Autodesk Fusion 360 part; units mm, degrees
(part 2 of 3)
  constraint coincident L1 L360.end
  constraint perpendicular L1 L360
  constraint midpoint L6 L361.start
  constraint coincident L3 L361.end
  constraint perpendicular L3 L361
  constraint equal L360 L361
  constraint midpoint L4 L362.start
  constraint perpendicular L2 L362
  constraint coincident L2 L362.end
  constraint coincident A356.centre L363.start
  constraint coincident L2 L363.end
  constraint perpendicular L2 L363
  constraint coincident L3 L364.end
  constraint perpendicular L3 L364
  constraint equal L363 L364
  constraint midpoint L2 L365.start
  constraint perpendicular L2 L365
  constraint midpoint L3 L366.start
  constraint perpendicular L3 L366
  constraint symmetric A356 L365 A357
  constraint symmetric A356 L366 A358
  constraint symmetric L366 A357 A359
  constraint equal A2 A52
  constraint equal A2 A3
  constraint tangent L5 A3
  constraint tangent L7 A3
  constraint tangent L5 A2
  constraint tangent L6 A2
  constraint vertical L7.start L59.start
  constraint tangent L4 A1
  constraint vertical A3.centre A53.centre
  constraint tangent L7 A1
  constraint tangent L6 A0
  constraint vertical A2.centre A52.centre
  constraint tangent L4 A0
  constraint horizontal L4
  constraint vertical L6
  constraint equal A0 A1
  constraint equal A1 A3
  constraint equal L6 L58
  constraint vertical A6.centre A60.centre
  constraint horizontal A3.centre A6.centre
  constraint horizontal A7.centre A10.centre
  constraint horizontal A11.centre A14.centre
  constraint horizontal A15.centre A18.centre
  constraint horizontal A19.centre A22.centre
  constraint horizontal A23.centre A26.centre
  constraint horizontal A27.centre A30.centre
  constraint horizontal A31.centre A34.centre
  constraint horizontal A35.centre A38.centre
  constraint horizontal A39.centre A42.centre
  constraint horizontal A43.centre A46.centre
  constraint horizontal A47.centre A50.centre
  constraint tangent L8 A4
  constraint tangent L10 A4
  constraint tangent L10 A6
  constraint tangent L9 A6
  constraint tangent L9 A7
  constraint tangent L11 A7
  constraint tangent L8 A5
  constraint tangent L11 A5
  constraint horizontal L8
  constraint vertical L10
  constraint horizontal L9
  constraint vertical L11
  constraint equal A4 A5
  constraint equal A6 A7
  constraint equal A4 A6
  constraint horizontal L12
  constraint vertical L14
  constraint horizontal L13
  constraint vertical L15
  constraint equal A8 A9
  constraint equal A8 A10
  constraint equal A10 A11
  constraint tangent L14 A10
  constraint tangent L13 A10
  constraint tangent L13 A11
  constraint tangent L15 A11
  constraint tangent L15 A9
  constraint tangent L12 A9
  constraint tangent L12 A8
  constraint tangent L14 A8
  constraint equal L8 L10
  constraint equal L12 L14
  constraint equal L16 L18
  constraint horizontal L16
  constraint vertical L18
  constraint horizontal L17
  constraint vertical L19
  constraint tangent L16 A13
  constraint tangent L19 A13
  constraint tangent L16 A12
  constraint tangent L18 A12
  constraint tangent L18 A14
  constraint tangent L17 A14
  constraint tangent L17 A15
  constraint tangent L19 A15
  constraint equal A12 A13
  constraint equal A12 A14
  constraint equal A14 A15
  constraint horizontal L20
  constraint horizontal L21
  constraint vertical L23
  constraint horizontal L24
  constraint vertical L26
  constraint vertical L22
  constraint horizontal L25
  constraint vertical L27
  constraint horizontal L28
  constraint vertical L30
  constraint vertical L31
  constraint horizontal L29
  constraint horizontal L32
  constraint horizontal L33
  constraint vertical L35
  constraint vertical L34
  constraint horizontal L36
  constraint horizontal L37
  constraint vertical L38
  constraint vertical L39
  constraint vertical L42
  constraint horizontal L40
  constraint vertical L43
  constraint horizontal L41
  constraint horizontal L45
  constraint vertical L46
  constraint horizontal L44
  constraint vertical L47
  constraint horizontal L48
  constraint vertical L50
  constraint horizontal L49
  constraint vertical L51
  constraint vertical L54
  constraint horizontal L52
  constraint vertical L55
  constraint horizontal L53
  constraint tangent L24 A20
  constraint tangent L26 A22
  constraint tangent L26 A20
  constraint tangent L25 A22
  constraint tangent L25 A23
  constraint tangent L24 A21
  constraint tangent L27 A21
  constraint tangent L27 A23
  constraint tangent L20 A16
  constraint tangent L22 A16
  constraint tangent L22 A18
  constraint tangent L21 A18
  constraint tangent L21 A19
  constraint tangent L23 A19
  constraint tangent L23 A17
  constraint tangent L20 A17
  constraint equal L20 L22
  constraint equal L24 L26
  constraint equal L28 L30
  constraint equal L32 L34
  constraint equal L36 L38
  constraint equal L40 L42
  constraint equal L44 L46
  constraint equal L48 L50
  constraint equal L52 L54
  constraint equal A16 A17
  constraint equal A16 A18
  constraint equal A17 A19
  constraint equal A20 A21
  constraint equal A21 A23
  constraint equal A22 A23
  constraint equal A24 A25
  constraint equal A25 A27
  constraint equal A26 A27
  constraint equal A26 A28
  constraint equal A28 A29
  constraint equal A29 A31
  constraint equal A30 A31
  constraint equal A30 A32
  constraint equal A32 A33
  constraint equal A33 A35
  constraint equal A34 A35
  constraint equal A34 A36
  constraint equal A36 A37
  constraint equal A37 A39
  constraint equal A38 A39
  constraint equal A38 A40
  constraint equal A40 A41
  constraint equal A41 A43
  constraint equal A42 A43
  constraint equal A42 A46
  constraint equal A44 A46
  constraint equal A44 A45
  constraint equal A45 A47
  constraint equal A47 A50
  constraint equal A48 A50
  constraint equal A48 A49
  constraint equal A49 A51
  constraint tangent L28 A24
  constraint tangent L30 A24
  constraint tangent L30 A26
  constraint tangent L29 A26
  constraint tangent L29 A27
  constraint tangent L31 A27
  constraint tangent L28 A25
  constraint tangent L31 A25
  constraint tangent L32 A28
  constraint tangent L34 A28
  constraint tangent L34 A30
  constraint tangent L33 A30
  constraint tangent L32 A29
  constraint tangent L35 A29
  constraint tangent L36 A32
  constraint tangent L38 A32
  constraint tangent L35 A31
  constraint tangent L38 A34
  constraint tangent L33 A31
  constraint tangent L37 A34
  constraint tangent L36 A33
  constraint tangent L39 A33
  constraint tangent L39 A35
  constraint tangent L37 A35
  constraint tangent L40 A36
  constraint tangent L42 A36
  constraint tangent L40 A37
  constraint tangent L43 A37
  constraint tangent L43 A39
  constraint tangent L41 A39
  constraint tangent L42 A38
  constraint tangent L41 A38
  constraint tangent L44 A40
  constraint tangent L44 A41
  constraint tangent L47 A41
  constraint tangent L47 A43
  constraint tangent L45 A43
  constraint tangent L46 A42
  constraint tangent L45 A42
  constraint tangent L46 A40
  constraint tangent L50 A46
  constraint tangent L49 A46
  constraint tangent L49 A47
  constraint tangent L51 A47
  constraint tangent L48 A44
  constraint tangent L50 A44
  constraint tangent L48 A45
  constraint tangent L51 A45
  constraint tangent L52 A48
  constraint tangent L54 A48
  constraint tangent L54 A50
  constraint tangent L53 A50
  constraint tangent L53 A51
  constraint tangent L55 A51
  constraint tangent L55 A49
  constraint tangent L52 A49
  constraint equal L8 L12
  constraint equal L12 L16
  constraint equal L16 L20
  constraint equal L20 L24
  constraint equal L24 L28
  constraint equal L28 L32
  constraint equal L32 L36
  constraint equal L36 L40
  constraint equal L40 L44
  constraint equal L44 L48
  constraint equal L48 L52
  constraint equal A5 A8
  constraint equal A9 A12
  constraint equal A13 A16
  constraint equal A17 A20
  constraint equal A1 A4
  constraint equal L7 L10
  constraint midpoint L11 L367.start
  constraint midpoint L14 L367.end
  constraint midpoint L15 L368.start
  constraint midpoint L18 L368.end
  constraint midpoint L19 L369.start
  constraint midpoint L22 L369.end
  constraint parallel L368 L369
  constraint midpoint L27 L370.start
  constraint midpoint L30 L370.end
  constraint midpoint L31 L371.start
  constraint midpoint L34 L371.end
  constraint midpoint L35 L372.start
  constraint midpoint L38 L372.end
  constraint midpoint L43 L373.start
  constraint midpoint L46 L373.end
  constraint midpoint L47 L374.start
  constraint midpoint L50 L374.end
  constraint midpoint L51 L375.start
  constraint midpoint L54 L375.end
  constraint equal L374 L375
  constraint equal L373 L374
  constraint equal L372 L373
  constraint midpoint L59 L376.start
  constraint midpoint L62 L376.end
  constraint equal L375 L376
  constraint equal L371 L372
  constraint equal L370 L371
  constraint equal L369 L370
  constraint equal L367 L368
  constraint equal L368 L376
  constraint midpoint L39 L377.start
  constraint midpoint L42 L377.end
  constraint midpoint L23 L378.start
  constraint midpoint L26 L378.end
  constraint equal L377 L378
  constraint equal A21 A24
  constraint horizontal L379
  constraint perpendicular L379 L380
  constraint parallel L379 L381
  constraint parallel L380 L382
  constraint coincident L383 P1
  constraint coincident L384 P1
  constraint equal L379 L382
  constraint midpoint L55 P2
  constraint horizontal P1 P2
  constraint coincident P1 P0
  constraint horizontal L360.start P5
  constraint midpoint L120 P4
  constraint vertical P5 P4
  constraint horizontal L385
  constraint perpendicular L385 L386
  constraint parallel L385 L387
  constraint parallel L386 L388
  constraint coincident L389 P5
  constraint coincident L390 P5
  constraint coincident P5 P3
  constraint equal L385 L388
  constraint midpoint L52 P6
  constraint vertical P1 P6
  constraint horizontal L391
  constraint perpendicular L391 L392
  constraint parallel L391 L393
  constraint parallel L392 L394
  constraint coincident L395 P7
  constraint coincident L396 P7
  constraint equal L379 L391
  constraint equal L391 L392
  constraint vertical L362.start P7
  constraint horizontal L361.start P7
  constraint midpoint L56 P8
  constraint midpoint L58 P9
  constraint horizontal L397
  constraint perpendicular L397 L398
  constraint parallel L397 L399
  constraint parallel L398 L400
  constraint coincident L401 P10
  constraint coincident L402 P10
  constraint vertical P8 P10
  constraint horizontal P9 P10
  constraint equal L397 L400
  constraint equal L393 L397
  measures "d28" distance of L0.start L2.end
  measures "d29" distance of L1.end L2.end
  measures "d32" diameter of A356
  measures "d33" distance of A356.centre L363.end
  measures "d35" distance of L0 L313
  measures "d39" distance of L379.start L379.end
  measures "d40" distance of L385.start L386.start
  measures "d41" distance of L382 L386
  measures "d42" distance of L393 L397
  measures "d43" diameter of A360
extrude "Extrude1" add sketch "plate-2026-01-07T20_54_01.375Z" along normal blind 1.5
fillet "Fillet1" radius 2.5 4 edges at (-11.2624, 12.475, 0.75) (-11.2624, -135.013, 0.75) (318.4436, -135.013, 0.75) (318.4436, 12.475, 0.75)
sketch "Sketch2" plane through (0, 0, 1.5) normal (0, 0, 1) x (-1, 0, 0)
  line L0 (-21.154, 19.2163) -> (-45.304, 19.2163) construction
  line L1 (-45.304, 19.2163) -> (-45.304, 5.2163) construction
  line L2 (-45.304, 5.2163) -> (-21.154, 5.2163) construction
  line L3 (-21.154, 5.2163) -> (-21.154, 19.2163) construction
  arc A0 (-88.75, 50.15) -> (-88.25, 50.65) centre (-88.75, 50.65) ccw
  line L4 (-88.75, 50.15) -> (-101.75, 50.15)
  arc A1 (-102.25, 50.65) -> (-101.75, 50.15) centre (-101.75, 50.65) ccw
  line L5 (-102.25, 50.65) -> (-102.25, 63.65)
  arc A2 (-101.75, 64.15) -> (-102.25, 63.65) centre (-101.75, 63.65) ccw
  line L6 (-101.75, 64.15) -> (-88.75, 64.15)
  arc A3 (-88.25, 63.65) -> (-88.75, 64.15) centre (-88.75, 63.65) ccw
  line L7 (-88.25, 63.65) -> (-88.25, 50.65)
  arc A4 (-269.7253, 7.287) -> (-269.2252, 7.787) centre (-269.7253, 7.787) ccw
  line L8 (-269.7253, 7.287) -> (-282.7252, 7.287)
  arc A5 (-283.2253, 7.787) -> (-282.7252, 7.287) centre (-282.7252, 7.787) ccw
  line L9 (-283.2253, 7.787) -> (-283.2253, 20.787)
  arc A6 (-282.7252, 21.287) -> (-283.2253, 20.787) centre (-282.7252, 20.787) ccw
  line L10 (-282.7252, 21.287) -> (-269.7253, 21.287)
  arc A7 (-269.2253, 20.787) -> (-269.7253, 21.287) centre (-269.7253, 20.787) ccw
  line L11 (-269.2253, 20.787) -> (-269.2252, 7.787)
  arc A8 (-107.8, 50.15) -> (-107.3, 50.65) centre (-107.8, 50.65) ccw
  line L12 (-107.8, 50.15) -> (-120.8, 50.15)
  arc A9 (-121.3, 50.65) -> (-120.8, 50.15) centre (-120.8, 50.65) ccw
  line L13 (-121.3, 50.65) -> (-121.3, 63.65)
  arc A10 (-120.8, 64.15) -> (-121.3, 63.65) centre (-120.8, 63.65) ccw
  line L14 (-120.8, 64.15) -> (-107.8, 64.15)
  arc A11 (-107.3, 63.65) -> (-107.8, 64.15) centre (-107.8, 63.65) ccw
  line L15 (-107.3, 63.65) -> (-107.3, 50.65)
  arc A12 (-207.8125, 69.2) -> (-207.3125, 69.7) centre (-207.8125, 69.7) ccw
  line L16 (-207.8125, 69.2) -> (-220.8125, 69.2)
  arc A13 (-221.3125, 69.7) -> (-220.8125, 69.2) centre (-220.8125, 69.7) ccw
  line L17 (-221.3125, 69.7) -> (-221.3125, 82.7)
  arc A14 (-220.8125, 83.2) -> (-221.3125, 82.7) centre (-220.8125, 82.7) ccw
  line L18 (-220.8125, 83.2) -> (-207.8125, 83.2)
  arc A15 (-207.3125, 82.7) -> (-207.8125, 83.2) centre (-207.8125, 82.7) ccw
  line L19 (-207.3125, 82.7) -> (-207.3125, 69.7)
  arc A16 (-203.05, 50.15) -> (-202.55, 50.65) centre (-203.05, 50.65) ccw
  line L20 (-203.05, 50.15) -> (-216.05, 50.15)
  arc A17 (-216.55, 50.65) -> (-216.05, 50.15) centre (-216.05, 50.65) ccw
  line L21 (-216.55, 50.65) -> (-216.55, 63.65)
  arc A18 (-216.05, 64.15) -> (-216.55, 63.65) centre (-216.05, 63.65) ccw
  line L22 (-216.05, 64.15) -> (-203.05, 64.15)
  arc A19 (-202.55, 63.65) -> (-203.05, 64.15) centre (-203.05, 63.65) ccw
  line L23 (-202.55, 63.65) -> (-202.55, 50.65)
  arc A20 (-6.4933, 89.25) -> (-5.9933, 89.75) centre (-6.4932, 89.75) ccw
  line L24 (-6.4933, 89.25) -> (-12.4932, 89.25)
  arc A21 (-12.9933, 89.75) -> (-12.4932, 89.25) centre (-12.4932, 89.75) ccw
  line L25 (-12.9932, 89.75) -> (-12.9933, 103.75)
  arc A22 (-12.4932, 104.25) -> (-12.9933, 103.75) centre (-12.4932, 103.75) ccw
  line L26 (-12.4932, 104.25) -> (-6.4932, 104.25)
  arc A23 (-5.9932, 103.75) -> (-6.4932, 104.25) centre (-6.4933, 103.75) ccw
  line L27 (-5.9932, 103.75) -> (-5.9933, 89.75)
  arc A24 (-291.1562, 31.1) -> (-290.6562, 31.6) centre (-291.1563, 31.6) ccw
  line L28 (-291.1562, 31.1) -> (-304.1562, 31.1)
  arc A25 (-304.6562, 31.6) -> (-304.1562, 31.1) centre (-304.1563, 31.6) ccw
  line L29 (-304.6562, 31.6) -> (-304.6562, 44.6)
  arc A26 (-304.1562, 45.1) -> (-304.6563, 44.6) centre (-304.1563, 44.6) ccw
  line L30 (-304.1562, 45.1) -> (-291.1562, 45.1)
  arc A27 (-290.6562, 44.6) -> (-291.1563, 45.1) centre (-291.1562, 44.6) ccw
  line L31 (-290.6562, 44.6) -> (-290.6562, 31.6)
  arc A28 (-188.7625, 69.2) -> (-188.2625, 69.7) centre (-188.7625, 69.7) ccw
  line L32 (-188.7625, 69.2) -> (-201.7625, 69.2)
  arc A29 (-202.2625, 69.7) -> (-201.7625, 69.2) centre (-201.7625, 69.7) ccw
  line L33 (-202.2625, 69.7) -> (-202.2625, 82.7)
  arc A30 (-201.7625, 83.2) -> (-202.2625, 82.7) centre (-201.7625, 82.7) ccw
  line L34 (-201.7625, 83.2) -> (-188.7625, 83.2)
  arc A31 (-188.2625, 82.7) -> (-188.7625, 83.2) centre (-188.7625, 82.7) ccw
  line L35 (-188.2625, 82.7) -> (-188.2625, 69.7)
  arc A32 (-36.3625, 69.2) -> (-35.8625, 69.7) centre (-36.3625, 69.7) ccw
  line L36 (-36.3625, 69.2) -> (-49.3625, 69.2)
  arc A33 (-49.8625, 69.7) -> (-49.3625, 69.2) centre (-49.3625, 69.7) ccw
  line L37 (-49.8625, 69.7) -> (-49.8625, 82.7)
  arc A34 (-49.3625, 83.2) -> (-49.8625, 82.7) centre (-49.3625, 82.7) ccw
  line L38 (-49.3625, 83.2) -> (-36.3625, 83.2)
  arc A35 (-35.8625, 82.7) -> (-36.3625, 83.2) centre (-36.3625, 82.7) ccw
  line L39 (-35.8625, 82.7) -> (-35.8625, 69.7)
  arc A36 (-169.7125, 69.2) -> (-169.2125, 69.7) centre (-169.7125, 69.7) ccw
  line L40 (-169.7125, 69.2) -> (-182.7125, 69.2)
  arc A37 (-183.2125, 69.7) -> (-182.7125, 69.2) centre (-182.7125, 69.7) ccw
  line L41 (-183.2125, 69.7) -> (-183.2125, 82.7)
  arc A38 (-182.7125, 83.2) -> (-183.2125, 82.7) centre (-182.7125, 82.7) ccw
  line L42 (-182.7125, 83.2) -> (-169.7125, 83.2)
  arc A39 (-169.2125, 82.7) -> (-169.7125, 83.2) centre (-169.7125, 82.7) ccw
  line L43 (-169.2125, 82.7) -> (-169.2125, 69.7)
  arc A40 (-164.9501, 7.287) -> (-164.4501, 7.787) centre (-164.9501, 7.787) ccw
  line L44 (-164.9501, 7.287) -> (-177.9501, 7.287)
  arc A41 (-178.4501, 7.787) -> (-177.9501, 7.287) centre (-177.9501, 7.787) ccw
  line L45 (-178.4501, 7.787) -> (-178.4501, 20.787)
  arc A42 (-177.9501, 21.287) -> (-178.4501, 20.787) centre (-177.9501, 20.787) ccw
  line L46 (-177.9501, 21.287) -> (-164.9501, 21.287)
  arc A43 (-164.4501, 20.787) -> (-164.9501, 21.287) centre (-164.9501, 20.787) ccw
  line L47 (-164.4501, 20.787) -> (-164.4501, 7.787)
  arc A44 (-212.575, 31.1) -> (-212.075, 31.6) centre (-212.575, 31.6) ccw
  line L48 (-212.575, 31.1) -> (-225.575, 31.1)
  arc A45 (-226.075, 31.6) -> (-225.575, 31.1) centre (-225.575, 31.6) ccw
  line L49 (-226.075, 31.6) -> (-226.075, 44.6)
  arc A46 (-225.575, 45.1) -> (-226.075, 44.6) centre (-225.575, 44.6) ccw
  line L50 (-225.575, 45.1) -> (-212.575, 45.1)
  arc A47 (-212.075, 44.6) -> (-212.575, 45.1) centre (-212.575, 44.6) ccw
  line L51 (-212.075, 44.6) -> (-212.075, 31.6)
  arc A48 (-275.638, 32.1) -> (-275.138, 32.6) centre (-275.638, 32.6) ccw
  line L52 (-275.638, 32.1) -> (-281.638, 32.1)
  arc A49 (-282.138, 32.6) -> (-281.638, 32.1) centre (-281.638, 32.6) ccw
  line L53 (-282.138, 32.6) -> (-282.138, 46.6)
  arc A50 (-281.638, 47.1) -> (-282.138, 46.6) centre (-281.638, 46.6) ccw
  line L54 (-281.638, 47.1) -> (-275.638, 47.1)
  arc A51 (-275.138, 46.6) -> (-275.638, 47.1) centre (-275.638, 46.6) ccw
  line L55 (-275.138, 46.6) -> (-275.138, 32.6)
  arc A52 (-260.2, 31.1) -> (-259.7, 31.6) centre (-260.2, 31.6) ccw
  line L56 (-260.2, 31.1) -> (-273.2, 31.1)
  arc A53 (-273.7, 31.6) -> (-273.2, 31.1) centre (-273.2, 31.6) ccw
  line L57 (-273.7, 31.6) -> (-273.7, 44.6)
  arc A54 (-273.2, 45.1) -> (-273.7, 44.6) centre (-273.2, 44.6) ccw
  line L58 (-273.2, 45.1) -> (-260.2, 45.1)
  arc A55 (-259.7, 44.6) -> (-260.2, 45.1) centre (-260.2, 44.6) ccw
  line L59 (-259.7, 44.6) -> (-259.7, 31.6)
  arc A56 (-243.5313, 88.25) -> (-243.0313, 88.75) centre (-243.5313, 88.75) ccw
  line L60 (-243.5313, 88.25) -> (-256.5313, 88.25)
  arc A57 (-257.0312, 88.75) -> (-256.5312, 88.25) centre (-256.5312, 88.75) ccw
  line L61 (-257.0312, 88.75) -> (-257.0313, 101.75)
  arc A58 (-256.5312, 102.25) -> (-257.0312, 101.75) centre (-256.5312, 101.75) ccw
  line L62 (-256.5312, 102.25) -> (-243.5312, 102.25)
  arc A59 (-243.0313, 101.75) -> (-243.5313, 102.25) centre (-243.5312, 101.75) ccw
  line L63 (-243.0312, 101.75) -> (-243.0312, 88.75)
  arc A60 (-83.9875, 88.25) -> (-83.4875, 88.75) centre (-83.9875, 88.75) ccw
  line L64 (-83.9875, 88.25) -> (-96.9875, 88.25)
  arc A61 (-97.4875, 88.75) -> (-96.9875, 88.25) centre (-96.9875, 88.75) ccw
  line L65 (-97.4875, 88.75) -> (-97.4875, 101.75)
  arc A62 (-96.9875, 102.25) -> (-97.4875, 101.75) centre (-96.9875, 101.75) ccw
  line L66 (-96.9875, 102.25) -> (-83.9875, 102.25)
  arc A63 (-83.4875, 101.75) -> (-83.9875, 102.25) centre (-83.9875, 101.75) ccw
  line L67 (-83.4875, 101.75) -> (-83.4875, 88.75)
  arc A64 (-93.5125, 69.2) -> (-93.0125, 69.7) centre (-93.5125, 69.7) ccw
  line L68 (-93.5125, 69.2) -> (-106.5125, 69.2)
  arc A65 (-107.0125, 69.7) -> (-106.5125, 69.2) centre (-106.5125, 69.7) ccw
  line L69 (-107.0125, 69.7) -> (-107.0125, 82.7)
  arc A66 (-106.5125, 83.2) -> (-107.0125, 82.7) centre (-106.5125, 82.7) ccw
  line L70 (-106.5125, 83.2) -> (-93.5125, 83.2)
  arc A67 (-93.0125, 82.7) -> (-93.5125, 83.2) centre (-93.5125, 82.7) ccw
  line L71 (-93.0125, 82.7) -> (-93.0125, 69.7)
  arc A68 (-270.9156, 107.3) -> (-270.4156, 107.8) centre (-270.9156, 107.8) ccw
  line L72 (-270.9156, 107.3) -> (-283.9156, 107.3)
  arc A69 (-284.4156, 107.8) -> (-283.9156, 107.3) centre (-283.9156, 107.8) ccw
  line L73 (-284.4156, 107.8) -> (-284.4156, 120.8)
  arc A70 (-283.9156, 121.3) -> (-284.4156, 120.8) centre (-283.9156, 120.8) ccw
  line L74 (-283.9156, 121.3) -> (-270.9156, 121.3)
  arc A71 (-270.4156, 120.8) -> (-270.9156, 121.3) centre (-270.9156, 120.8) ccw
  line L75 (-270.4156, 120.8) -> (-270.4156, 107.8)
  arc A72 (-45.8875, 88.25) -> (-45.3875, 88.75) centre (-45.8875, 88.75) ccw
  line L76 (-45.8875, 88.25) -> (-58.8875, 88.25)
  arc A73 (-59.3875, 88.75) -> (-58.8875, 88.25) centre (-58.8875, 88.75) ccw
  line L77 (-59.3875, 88.75) -> (-59.3875, 101.75)
  arc A74 (-58.8875, 102.25) -> (-59.3875, 101.75) centre (-58.8875, 101.75) ccw
  line L78 (-58.8875, 102.25) -> (-45.8875, 102.25)
  arc A75 (-45.3875, 101.75) -> (-45.8875, 102.25) centre (-45.8875, 101.75) ccw
  line L79 (-45.3875, 101.75) -> (-45.3875, 88.75)
  arc A76 (-77.9688, 108.3) -> (-77.4687, 108.8) centre (-77.9688, 108.8) ccw
  line L80 (-77.9688, 108.3) -> (-83.9688, 108.3)
  arc A77 (-84.4688, 108.8) -> (-83.9688, 108.3) centre (-83.9687, 108.8) ccw
  line L81 (-84.4688, 108.8) -> (-84.4687, 122.8)
  arc A78 (-83.9688, 123.3) -> (-84.4687, 122.8) centre (-83.9688, 122.8) ccw
  line L82 (-83.9688, 123.3) -> (-77.9688, 123.3)
  arc A79 (-77.4688, 122.8) -> (-77.9688, 123.3) centre (-77.9688, 122.8) ccw
  line L83 (-77.4688, 122.8) -> (-77.4687, 108.8)
  arc A80 (-251.762, 32.1) -> (-251.262, 32.6) centre (-251.762, 32.6) ccw
  line L84 (-251.762, 32.1) -> (-257.762, 32.1)
  arc A81 (-258.262, 32.6) -> (-257.762, 32.1) centre (-257.762, 32.6) ccw
  line L85 (-258.262, 32.6) -> (-258.262, 46.6)
  arc A82 (-257.762, 47.1) -> (-258.262, 46.6) centre (-257.762, 46.6) ccw
  line L86 (-257.762, 47.1) -> (-251.762, 47.1)
  arc A83 (-251.262, 46.6) -> (-251.762, 47.1) centre (-251.762, 46.6) ccw
  line L87 (-251.262, 46.6) -> (-251.262, 32.6)
  arc A84 (-231.6252, 7.287) -> (-231.1252, 7.787) centre (-231.6252, 7.787) ccw
  line L88 (-231.6252, 7.287) -> (-244.6252, 7.287)
  arc A85 (-245.1252, 7.787) -> (-244.6252, 7.287) centre (-244.6252, 7.787) ccw
  line L89 (-245.1252, 7.787) -> (-245.1252, 20.787)
  arc A86 (-244.6252, 21.287) -> (-245.1252, 20.787) centre (-244.6252, 20.787) ccw
  line L90 (-244.6252, 21.287) -> (-231.6253, 21.287)
  arc A87 (-231.1252, 20.787) -> (-231.6253, 21.287) centre (-231.6253, 20.787) ccw
  line L91 (-231.1252, 20.787) -> (-231.1252, 7.787)
  arc A88 (-198.2875, 88.25) -> (-197.7875, 88.75) centre (-198.2875, 88.75) ccw
  line L92 (-198.2875, 88.25) -> (-211.2875, 88.25)
  arc A89 (-211.7875, 88.75) -> (-211.2875, 88.25) centre (-211.2875, 88.75) ccw
  line L93 (-211.7875, 88.75) -> (-211.7875, 101.75)
  arc A90 (-211.2875, 102.25) -> (-211.7875, 101.75) centre (-211.2875, 101.75) ccw
  line L94 (-211.2875, 102.25) -> (-198.2875, 102.25)
  arc A91 (-197.7875, 101.75) -> (-198.2875, 102.25) centre (-198.2875, 101.75) ccw
  line L95 (-197.7875, 101.75) -> (-197.7875, 88.75)
  arc A92 (-222.1, 50.15) -> (-221.6, 50.65) centre (-222.1, 50.65) ccw
  line L96 (-222.1, 50.15) -> (-235.1, 50.15)
  arc A93 (-235.6, 50.65) -> (-235.1, 50.15) centre (-235.1, 50.65) ccw
  line L97 (-235.6, 50.65) -> (-235.6, 63.65)
  arc A94 (-235.1, 64.15) -> (-235.6, 63.65) centre (-235.1, 63.65) ccw
  line L98 (-235.1, 64.15) -> (-222.1, 64.15)
  arc A95 (-221.6, 63.65) -> (-222.1, 64.15) centre (-222.1, 63.65) ccw
  line L99 (-221.6, 63.65) -> (-221.6, 50.65)
  arc A96 (-291.1563, 69.2) -> (-290.6563, 69.7) centre (-291.1563, 69.7) ccw
  line L100 (-291.1562, 69.2) -> (-304.1562, 69.2)
  arc A97 (-304.6562, 69.7) -> (-304.1563, 69.2) centre (-304.1563, 69.7) ccw
  line L101 (-304.6562, 69.7) -> (-304.6562, 82.7)
  arc A98 (-304.1562, 83.2) -> (-304.6562, 82.7) centre (-304.1562, 82.7) ccw
  line L102 (-304.1562, 83.2) -> (-291.1562, 83.2)
  arc A99 (-290.6562, 82.7) -> (-291.1562, 83.2) centre (-291.1562, 82.7) ccw
  line L103 (-290.6562, 82.7) -> (-290.6563, 69.7)
  arc A100 (-22.075, 31.1) -> (-21.575, 31.6) centre (-22.075, 31.6) ccw
  line L104 (-22.075, 31.1) -> (-35.075, 31.1)
  arc A101 (-35.575, 31.6) -> (-35.075, 31.1) centre (-35.075, 31.6) ccw
  line L105 (-35.575, 31.6) -> (-35.575, 44.6)
  arc A102 (-35.075, 45.1) -> (-35.575, 44.6) centre (-35.075, 44.6) ccw
  line L106 (-35.075, 45.1) -> (-22.075, 45.1)
  arc A103 (-21.575, 44.6) -> (-22.075, 45.1) centre (-22.075, 44.6) ccw
  line L107 (-21.575, 44.6) -> (-21.575, 31.6)
  arc A104 (-145.9, 50.15) -> (-145.4, 50.65) centre (-145.9, 50.65) ccw
  line L108 (-145.9, 50.15) -> (-158.9, 50.15)
  arc A105 (-159.4, 50.65) -> (-158.9, 50.15) centre (-158.9, 50.65) ccw
  line L109 (-159.4, 50.65) -> (-159.4, 63.65)
  arc A106 (-158.9, 64.15) -> (-159.4, 63.65) centre (-158.9, 63.65) ccw
  line L110 (-158.9, 64.15) -> (-145.9, 64.15)
  arc A107 (-145.4, 63.65) -> (-145.9, 64.15) centre (-145.9, 63.65) ccw
  line L111 (-145.4, 63.65) -> (-145.4, 50.65)
  arc A108 (-69.7, 50.15) -> (-69.2, 50.65) centre (-69.7, 50.65) ccw
  line L112 (-69.7, 50.15) -> (-82.7, 50.15)
  arc A109 (-83.2, 50.65) -> (-82.7, 50.15) centre (-82.7, 50.65) ccw
  line L113 (-83.2, 50.65) -> (-83.2, 63.65)
  arc A110 (-82.7, 64.15) -> (-83.2, 63.65) centre (-82.7, 63.65) ccw
  line L114 (-82.7, 64.15) -> (-69.7, 64.15)
  arc A111 (-69.2, 63.65) -> (-69.7, 64.15) centre (-69.7, 63.65) ccw
  line L115 (-69.2, 63.65) -> (-69.2, 50.65)
  arc A112 (-231.625, 107.3) -> (-231.125, 107.8) centre (-231.625, 107.8) ccw
  line L116 (-231.625, 107.3) -> (-244.625, 107.3)
  arc A113 (-245.125, 107.8) -> (-244.625, 107.3) centre (-244.625, 107.8) ccw
  line L117 (-245.125, 107.8) -> (-245.125, 120.8)
  arc A114 (-244.625, 121.3) -> (-245.125, 120.8) centre (-244.625, 120.8) ccw
  line L118 (-244.625, 121.3) -> (-231.625, 121.3)
  arc A115 (-231.125, 120.8) -> (-231.625, 121.3) centre (-231.625, 120.8) ccw
  line L119 (-231.125, 120.8) -> (-231.125, 107.8)
  arc A116 (-155.425, 31.1) -> (-154.925, 31.6) centre (-155.425, 31.6) ccw
  line L120 (-155.425, 31.1) -> (-168.425, 31.1)
  arc A117 (-168.925, 31.6) -> (-168.425, 31.1) centre (-168.425, 31.6) ccw
  line L121 (-168.925, 31.6) -> (-168.925, 44.6)
  arc A118 (-168.425, 45.1) -> (-168.925, 44.6) centre (-168.425, 44.6) ccw
  line L122 (-168.425, 45.1) -> (-155.425, 45.1)
  arc A119 (-154.925, 44.6) -> (-155.425, 45.1) centre (-155.425, 44.6) ccw
  line L123 (-154.925, 44.6) -> (-154.925, 31.6)
  arc A120 (-103.0375, 88.25) -> (-102.5375, 88.75) centre (-103.0375, 88.75) ccw
  line L124 (-103.0375, 88.25) -> (-116.0375, 88.25)
  arc A121 (-116.5375, 88.75) -> (-116.0375, 88.25) centre (-116.0375, 88.75) ccw
  line L125 (-116.5375, 88.75) -> (-116.5375, 101.75)
  arc A122 (-116.0375, 102.25) -> (-116.5375, 101.75) centre (-116.0375, 101.75) ccw
  line L126 (-116.0375, 102.25) -> (-103.0375, 102.25)
  arc A123 (-102.5375, 101.75) -> (-103.0375, 102.25) centre (-103.0375, 101.75) ccw
  line L127 (-102.5375, 101.75) -> (-102.5375, 88.75)
  arc A124 (-177.9688, 108.3) -> (-177.4687, 108.8) centre (-177.9688, 108.8) ccw
  line L128 (-177.9688, 108.3) -> (-183.9688, 108.3)
  arc A125 (-184.4688, 108.8) -> (-183.9688, 108.3) centre (-183.9688, 108.8) ccw
  line L129 (-184.4688, 108.8) -> (-184.4688, 122.8)
  arc A126 (-183.9688, 123.3) -> (-184.4687, 122.8) centre (-183.9687, 122.8) ccw
  line L130 (-183.9688, 123.3) -> (-177.9688, 123.3)
  arc A127 (-177.4688, 122.8) -> (-177.9688, 123.3) centre (-177.9688, 122.8) ccw
  line L131 (-177.4688, 122.8) -> (-177.4687, 108.8)
  arc A128 (-79.225, 31.1) -> (-78.725, 31.6) centre (-79.225, 31.6) ccw
  line L132 (-79.225, 31.1) -> (-92.225, 31.1)
  arc A129 (-92.725, 31.6) -> (-92.225, 31.1) centre (-92.225, 31.6) ccw
  line L133 (-92.725, 31.6) -> (-92.725, 44.6)
  arc A130 (-92.225, 45.1) -> (-92.725, 44.6) centre (-92.225, 44.6) ccw
  line L134 (-92.225, 45.1) -> (-79.225, 45.1)
  arc A131 (-78.725, 44.6) -> (-79.225, 45.1) centre (-79.225, 44.6) ccw
  line L135 (-78.725, 44.6) -> (-78.725, 31.6)
  arc A132 (-273.2568, 70.2) -> (-272.7568, 70.7) centre (-273.2568, 70.7) ccw
  line L136 (-273.2568, 70.2) -> (-279.2568, 70.2)
  arc A133 (-279.7568, 70.7) -> (-279.2568, 70.2) centre (-279.2568, 70.7) ccw
  line L137 (-279.7568, 70.7) -> (-279.7568, 84.7)
  arc A134 (-279.2568, 85.2) -> (-279.7568, 84.7) centre (-279.2568, 84.7) ccw
  line L138 (-279.2568, 85.2) -> (-273.2568, 85.2)
  arc A135 (-272.7568, 84.7) -> (-273.2568, 85.2) centre (-273.2568, 84.7) ccw
  line L139 (-272.7568, 84.7) -> (-272.7568, 70.7)
  arc A136 (-29.2188, 107.3) -> (-28.7187, 107.8) centre (-29.2188, 107.8) ccw
  line L140 (-29.2188, 107.3) -> (-42.2188, 107.3)
  arc A137 (-42.7188, 107.8) -> (-42.2188, 107.3) centre (-42.2188, 107.8) ccw
  line L141 (-42.7188, 107.8) -> (-42.7188, 120.8)
  arc A138 (-42.2188, 121.3) -> (-42.7188, 120.8) centre (-42.2187, 120.8) ccw
  line L142 (-42.2188, 121.3) -> (-29.2188, 121.3)
  arc A139 (-28.7188, 120.8) -> (-29.2188, 121.3) centre (-29.2187, 120.8) ccw
  line L143 (-28.7188, 120.8) -> (-28.7187, 107.8)
  arc A140 (-122.0875, 88.25) -> (-121.5875, 88.75) centre (-122.0875, 88.75) ccw
  line L144 (-122.0875, 88.25) -> (-135.0875, 88.25)
  arc A141 (-135.5875, 88.75) -> (-135.0875, 88.25) centre (-135.0875, 88.75) ccw
  line L145 (-135.5875, 88.75) -> (-135.5875, 101.75)
  arc A142 (-135.0875, 102.25) -> (-135.5875, 101.75) centre (-135.0875, 101.75) ccw
  line L146 (-135.0875, 102.25) -> (-122.0875, 102.25)
  arc A143 (-121.5875, 101.75) -> (-122.0875, 102.25) centre (-122.0875, 101.75) ccw
  line L147 (-121.5875, 101.75) -> (-121.5875, 88.75)
  arc A144 (-3.025, 7.287) -> (-2.525, 7.787) centre (-3.025, 7.787) ccw
  line L148 (-3.025, 7.287) -> (-16.025, 7.287)
  arc A145 (-16.525, 7.787) -> (-16.025, 7.287) centre (-16.025, 7.787) ccw
  line L149 (-16.525, 7.787) -> (-16.525, 20.787)
  arc A146 (-16.025, 21.287) -> (-16.525, 20.787) centre (-16.025, 20.787) ccw
  line L150 (-16.025, 21.287) -> (-3.025, 21.287)
  arc A147 (-2.525, 20.787) -> (-3.025, 21.287) centre (-3.025, 20.787) ccw
  line L151 (-2.525, 20.787) -> (-2.525, 7.787)
  arc A148 (-30.3693, 89.25) -> (-29.8693, 89.75) centre (-30.3692, 89.75) ccw
  line L152 (-30.3693, 89.25) -> (-36.3692, 89.25)
  arc A149 (-36.8693, 89.75) -> (-36.3692, 89.25) centre (-36.3692, 89.75) ccw
  line L153 (-36.8693, 89.75) -> (-36.8693, 103.75)
  arc A150 (-36.3693, 104.25) -> (-36.8693, 103.75) centre (-36.3693, 103.75) ccw
  line L154 (-36.3693, 104.25) -> (-30.3693, 104.25)
  arc A151 (-29.8693, 103.75) -> (-30.3693, 104.25) centre (-30.3693, 103.75) ccw
  line L155 (-29.8693, 103.75) -> (-29.8693, 89.75)
  arc A152 (-184, 50.15) -> (-183.5, 50.65) centre (-184, 50.65) ccw
  line L156 (-184, 50.15) -> (-197, 50.15)
  arc A153 (-197.5, 50.65) -> (-197, 50.15) centre (-197, 50.65) ccw
  line L157 (-197.5, 50.65) -> (-197.5, 63.65)
  arc A154 (-197, 64.15) -> (-197.5, 63.65) centre (-197, 63.65) ccw
  line L158 (-197, 64.15) -> (-184, 64.15)
  arc A155 (-183.5, 63.65) -> (-184, 64.15) centre (-184, 63.65) ccw
  line L159 (-183.5, 63.65) -> (-183.5, 50.65)
  arc A156 (-3.025, 31.1) -> (-2.525, 31.6) centre (-3.025, 31.6) ccw
  line L160 (-3.025, 31.1) -> (-16.025, 31.1)
  arc A157 (-16.525, 31.6) -> (-16.025, 31.1) centre (-16.025, 31.6) ccw
  line L161 (-16.525, 31.6) -> (-16.525, 44.6)
  arc A158 (-16.025, 45.1) -> (-16.525, 44.6) centre (-16.025, 44.6) ccw
  line L162 (-16.025, 45.1) -> (-3.025, 45.1)
  arc A159 (-2.525, 44.6) -> (-3.025, 45.1) centre (-3.025, 44.6) ccw
  line L163 (-2.525, 44.6) -> (-2.525, 31.6)
  arc A160 (-264.9625, 50.15) -> (-264.4625, 50.65) centre (-264.9625, 50.65) ccw
  line L164 (-264.9625, 50.15) -> (-277.9625, 50.15)
  arc A161 (-278.4625, 50.65) -> (-277.9625, 50.15) centre (-277.9625, 50.65) ccw
  line L165 (-278.4625, 50.65) -> (-278.4625, 63.65)
  arc A162 (-277.9625, 64.15) -> (-278.4625, 63.65) centre (-277.9625, 63.65) ccw
  line L166 (-277.9625, 64.15) -> (-264.9625, 64.15)
  arc A163 (-264.4625, 63.65) -> (-264.9625, 64.15) centre (-264.9625, 63.65) ccw
  line L167 (-264.4625, 63.65) -> (-264.4625, 50.65)
  arc A164 (-179.2375, 88.25) -> (-178.7375, 88.75) centre (-179.2375, 88.75) ccw
  line L168 (-179.2375, 88.25) -> (-192.2375, 88.25)
  arc A165 (-192.7375, 88.75) -> (-192.2375, 88.25) centre (-192.2375, 88.75) ccw
  line L169 (-192.7375, 88.75) -> (-192.7375, 101.75)
  arc A166 (-192.2375, 102.25) -> (-192.7375, 101.75) centre (-192.2375, 101.75) ccw
  line L170 (-192.2375, 102.25) -> (-179.2375, 102.25)
  arc A167 (-178.7375, 101.75) -> (-179.2375, 102.25) centre (-179.2375, 101.75) ccw
  line L171 (-178.7375, 101.75) -> (-178.7375, 88.75)
  arc A168 (-41.125, 7.287) -> (-40.625, 7.787) centre (-41.125, 7.787) ccw
  line L172 (-41.125, 7.287) -> (-54.125, 7.287)
  arc A169 (-54.625, 7.787) -> (-54.125, 7.287) centre (-54.125, 7.787) ccw
  line L173 (-54.625, 7.787) -> (-54.625, 20.787)
  arc A170 (-54.125, 21.287) -> (-54.625, 20.787) centre (-54.125, 20.787) ccw
  line L174 (-54.125, 21.287) -> (-41.125, 21.287)
  arc A171 (-40.625, 20.787) -> (-41.125, 21.287) centre (-41.125, 20.787) ccw
  line L175 (-40.625, 20.787) -> (-40.625, 7.787)
  arc A172 (-249.3808, 70.2) -> (-248.8807, 70.7) centre (-249.3808, 70.7) ccw
  line L176 (-249.3808, 70.2) -> (-255.3808, 70.2)
  arc A173 (-255.8808, 70.7) -> (-255.3808, 70.2) centre (-255.3808, 70.7) ccw
  line L177 (-255.8808, 70.7) -> (-255.8808, 84.7)
  arc A174 (-255.3808, 85.2) -> (-255.8808, 84.7) centre (-255.3808, 84.7) ccw
  line L178 (-255.3808, 85.2) -> (-249.3808, 85.2)
  arc A175 (-248.8808, 84.7) -> (-249.3808, 85.2) centre (-249.3808, 84.7) ccw
  line L179 (-248.8808, 84.7) -> (-248.8807, 70.7)
  arc A176 (-98.275, 7.287) -> (-97.775, 7.787) centre (-98.275, 7.787) ccw
  line L180 (-98.275, 7.287) -> (-111.275, 7.287)
  arc A177 (-111.775, 7.787) -> (-111.275, 7.287) centre (-111.275, 7.787) ccw
  line L181 (-111.775, 7.787) -> (-111.775, 20.787)
  arc A178 (-111.275, 21.287) -> (-111.775, 20.787) centre (-111.275, 20.787) ccw
  line L182 (-111.275, 21.287) -> (-98.275, 21.287)
  arc A179 (-97.775, 20.787) -> (-98.275, 21.287) centre (-98.275, 20.787) ccw
  line L183 (-97.775, 20.787) -> (-97.775, 7.787)
  arc A180 (-212.575, 107.3) -> (-212.075, 107.8) centre (-212.575, 107.8) ccw
  line L184 (-212.575, 107.3) -> (-225.575, 107.3)
  arc A181 (-226.075, 107.8) -> (-225.575, 107.3) centre (-225.575, 107.8) ccw
  line L185 (-226.075, 107.8) -> (-226.075, 120.8)
  arc A182 (-225.575, 121.3) -> (-226.075, 120.8) centre (-225.575, 120.8) ccw
  line L186 (-225.575, 121.3) -> (-212.575, 121.3)
  arc A183 (-212.075, 120.8) -> (-212.575, 121.3) centre (-212.575, 120.8) ccw
  line L187 (-212.075, 120.8) -> (-212.075, 107.8)
  arc A184 (-5.4063, 107.3) -> (-4.9062, 107.8) centre (-5.4063, 107.8) ccw
  line L188 (-5.4062, 107.3) -> (-18.4063, 107.3)
  arc A185 (-18.9062, 107.8) -> (-18.4063, 107.3) centre (-18.4062, 107.8) ccw
  line L189 (-18.9062, 107.8) -> (-18.9063, 120.8)
  arc A186 (-18.4062, 121.3) -> (-18.9063, 120.8) centre (-18.4062, 120.8) ccw
  line L190 (-18.4062, 121.3) -> (-5.4063, 121.3)
  arc A187 (-4.9062, 120.8) -> (-5.4063, 121.3) centre (-5.4063, 120.8) ccw
  line L191 (-4.9062, 120.8) -> (-4.9062, 107.8)
  arc A188 (-250.675, 107.3) -> (-250.175, 107.8) centre (-250.675, 107.8) ccw
  line L192 (-250.675, 107.3) -> (-263.675, 107.3)
  arc A189 (-264.175, 107.8) -> (-263.675, 107.3) centre (-263.675, 107.8) ccw
  line L193 (-264.175, 107.8) -> (-264.175, 120.8)
  arc A190 (-263.675, 121.3) -> (-264.175, 120.8) centre (-263.675, 120.8) ccw
  line L194 (-263.675, 121.3) -> (-250.675, 121.3)
  arc A191 (-250.175, 120.8) -> (-250.675, 121.3) centre (-250.675, 120.8) ccw
  line L195 (-250.175, 120.8) -> (-250.175, 107.8)
  arc A192 (-112.5625, 69.2) -> (-112.0625, 69.7) centre (-112.5625, 69.7) ccw
  line L196 (-112.5625, 69.2) -> (-125.5625, 69.2)
  arc A193 (-126.0625, 69.7) -> (-125.5625, 69.2) centre (-125.5625, 69.7) ccw
  line L197 (-126.0625, 69.7) -> (-126.0625, 82.7)
  arc A194 (-125.5625, 83.2) -> (-126.0625, 82.7) centre (-125.5625, 82.7) ccw
  line L198 (-125.5625, 83.2) -> (-112.5625, 83.2)
  arc A195 (-112.0625, 82.7) -> (-112.5625, 83.2) centre (-112.5625, 82.7) ccw
  line L199 (-112.0625, 82.7) -> (-112.0625, 69.7)
  arc A196 (-217.3375, 88.25) -> (-216.8375, 88.75) centre (-217.3375, 88.75) ccw
  line L200 (-217.3375, 88.25) -> (-230.3375, 88.25)
  arc A197 (-230.8375, 88.75) -> (-230.3375, 88.25) centre (-230.3375, 88.75) ccw
  line L201 (-230.8375, 88.75) -> (-230.8375, 101.75)
  arc A198 (-230.3375, 102.25) -> (-230.8375, 101.75) centre (-230.3375, 101.75) ccw
  line L202 (-230.3375, 102.25) -> (-217.3375, 102.25)
  arc A199 (-216.8375, 101.75) -> (-217.3375, 102.25) centre (-217.3375, 101.75) ccw
  line L203 (-216.8375, 101.75) -> (-216.8375, 88.75)
  arc A200 (-64.9375, 88.25) -> (-64.4375, 88.75) centre (-64.9375, 88.75) ccw
  line L204 (-64.9375, 88.25) -> (-77.9375, 88.25)
  arc A201 (-78.4375, 88.75) -> (-77.9375, 88.25) centre (-77.9375, 88.75) ccw
  line L205 (-78.4375, 88.75) -> (-78.4375, 101.75)
  arc A202 (-77.9375, 102.25) -> (-78.4375, 101.75) centre (-77.9375, 101.75) ccw
  line L206 (-77.9375, 102.25) -> (-64.9375, 102.25)
  arc A203 (-64.4375, 101.75) -> (-64.9375, 102.25) centre (-64.9375, 101.75) ccw
  line L207 (-64.4375, 101.75) -> (-64.4375, 88.75)
  arc A204 (-226.8625, 69.2) -> (-226.3625, 69.7) centre (-226.8625, 69.7) ccw
  line L208 (-226.8625, 69.2) -> (-239.8625, 69.2)
  arc A205 (-240.3625, 69.7) -> (-239.8625, 69.2) centre (-239.8625, 69.7) ccw
  line L209 (-240.3625, 69.7) -> (-240.3625, 82.7)
  arc A206 (-239.8625, 83.2) -> (-240.3625, 82.7) centre (-239.8625, 82.7) ccw
  line L210 (-239.8625, 83.2) -> (-226.8625, 83.2)
  arc A207 (-226.3625, 82.7) -> (-226.8625, 83.2) centre (-226.8625, 82.7) ccw
  line L211 (-226.3625, 82.7) -> (-226.3625, 69.7)
  arc A208 (-60.175, 7.287) -> (-59.675, 7.787) centre (-60.175, 7.787) ccw
  line L212 (-60.175, 7.287) -> (-73.175, 7.287)
  arc A209 (-73.675, 7.787) -> (-73.175, 7.287) centre (-73.175, 7.787) ccw
  line L213 (-73.675, 7.787) -> (-73.675, 20.787)
  arc A210 (-73.175, 21.287) -> (-73.675, 20.787) centre (-73.175, 20.787) ccw
  line L214 (-73.175, 21.287) -> (-60.175, 21.287)
  arc A211 (-59.675, 20.787) -> (-60.175, 21.287) centre (-60.175, 20.787) ccw
  line L215 (-59.675, 20.787) -> (-59.675, 7.787)
  arc A212 (-291.1563, 50.15) -> (-290.6563, 50.65) centre (-291.1563, 50.65) ccw
  line L216 (-291.1562, 50.15) -> (-304.1562, 50.15)
  arc A213 (-304.6562, 50.65) -> (-304.1562, 50.15) centre (-304.1563, 50.65) ccw
  line L217 (-304.6562, 50.65) -> (-304.6562, 63.65)
  arc A214 (-304.1562, 64.15) -> (-304.6562, 63.65) centre (-304.1563, 63.65) ccw
  line L218 (-304.1562, 64.15) -> (-291.1562, 64.15)
  arc A215 (-290.6562, 63.65) -> (-291.1563, 64.15) centre (-291.1562, 63.65) ccw
  line L219 (-290.6562, 63.65) -> (-290.6563, 50.65)
  arc A216 (-141.1375, 88.25) -> (-140.6375, 88.75) centre (-141.1375, 88.75) ccw
  line L220 (-141.1375, 88.25) -> (-154.1375, 88.25)
  arc A217 (-154.6375, 88.75) -> (-154.1375, 88.25) centre (-154.1375, 88.75) ccw
  line L221 (-154.6375, 88.75) -> (-154.6375, 101.75)
  arc A218 (-154.1375, 102.25) -> (-154.6375, 101.75) centre (-154.1375, 101.75) ccw
  line L222 (-154.1375, 102.25) -> (-141.1375, 102.25)
  arc A219 (-140.6375, 101.75) -> (-141.1375, 102.25) centre (-141.1375, 101.75) ccw
  line L223 (-140.6375, 101.75) -> (-140.6375, 88.75)
  arc A220 (-31.6, 50.15) -> (-31.1, 50.65) centre (-31.6, 50.65) ccw
  line L224 (-31.6, 50.15) -> (-44.6, 50.15)
  arc A221 (-45.1, 50.65) -> (-44.6, 50.15) centre (-44.6, 50.65) ccw
  line L225 (-45.1, 50.65) -> (-45.1, 63.65)
  arc A222 (-44.6, 64.15) -> (-45.1, 63.65) centre (-44.6, 63.65) ccw
  line L226 (-44.6, 64.15) -> (-31.6, 64.15)
  arc A223 (-31.1, 63.65) -> (-31.6, 64.15) centre (-31.6, 63.65) ccw
  line L227 (-31.1, 63.65) -> (-31.1, 50.65)
  arc A224 (-160.1875, 88.25) -> (-159.6875, 88.75) centre (-160.1875, 88.75) ccw
  line L228 (-160.1875, 88.25) -> (-173.1875, 88.25)
  arc A225 (-173.6875, 88.75) -> (-173.1875, 88.25) centre (-173.1875, 88.75) ccw
  line L229 (-173.6875, 88.75) -> (-173.6875, 101.75)
  arc A226 (-173.1875, 102.25) -> (-173.6875, 101.75) centre (-173.1875, 101.75) ccw
  line L230 (-173.1875, 102.25) -> (-160.1875, 102.25)
  arc A227 (-159.6875, 101.75) -> (-160.1875, 102.25) centre (-160.1875, 101.75) ccw
  line L231 (-159.6875, 101.75) -> (-159.6875, 88.75)
  arc A228 (-174.475, 31.1) -> (-173.975, 31.6) centre (-174.475, 31.6) ccw
  line L232 (-174.475, 31.1) -> (-187.475, 31.1)
  arc A229 (-187.975, 31.6) -> (-187.475, 31.1) centre (-187.475, 31.6) ccw
  line L233 (-187.975, 31.6) -> (-187.975, 44.6)
  arc A230 (-187.475, 45.1) -> (-187.975, 44.6) centre (-187.475, 44.6) ccw
  line L234 (-187.475, 45.1) -> (-174.475, 45.1)
  arc A231 (-173.975, 44.6) -> (-174.475, 45.1) centre (-174.475, 44.6) ccw
  line L235 (-173.975, 44.6) -> (-173.975, 31.6)
  arc A232 (-193.525, 107.3) -> (-193.025, 107.8) centre (-193.525, 107.8) ccw
  line L236 (-193.525, 107.3) -> (-206.525, 107.3)
  arc A233 (-207.025, 107.8) -> (-206.525, 107.3) centre (-206.525, 107.8) ccw
  line L237 (-207.025, 107.8) -> (-207.025, 120.8)
  arc A234 (-206.525, 121.3) -> (-207.025, 120.8) centre (-206.525, 120.8) ccw
  line L238 (-206.525, 121.3) -> (-193.525, 121.3)
  arc A235 (-193.025, 120.8) -> (-193.525, 121.3) centre (-193.525, 120.8) ccw
  line L239 (-193.025, 120.8) -> (-193.025, 107.8)
  arc A236 (-257.8188, 69.2) -> (-257.3187, 69.7) centre (-257.8188, 69.7) ccw
  line L240 (-257.8188, 69.2) -> (-270.8188, 69.2)
  arc A237 (-271.3188, 69.7) -> (-270.8188, 69.2) centre (-270.8188, 69.7) ccw
  line L241 (-271.3188, 69.7) -> (-271.3187, 82.7)
  arc A238 (-270.8188, 83.2) -> (-271.3188, 82.7) centre (-270.8188, 82.7) ccw
  line L242 (-270.8188, 83.2) -> (-257.8188, 83.2)
  arc A239 (-257.3188, 82.7) -> (-257.8188, 83.2) centre (-257.8188, 82.7) ccw
  line L243 (-257.3188, 82.7) -> (-257.3187, 69.7)
  arc A240 (-14.9313, 88.25) -> (-14.4313, 88.75) centre (-14.9312, 88.75) ccw
  line L244 (-14.9313, 88.25) -> (-27.9312, 88.25)
  arc A241 (-28.4313, 88.75) -> (-27.9312, 88.25) centre (-27.9312, 88.75) ccw
  line L245 (-28.4313, 88.75) -> (-28.4313, 101.75)
  arc A242 (-27.9312, 102.25) -> (-28.4313, 101.75) centre (-27.9312, 101.75) ccw
  line L246 (-27.9312, 102.25) -> (-14.9313, 102.25)
  arc A243 (-14.4313, 101.75) -> (-14.9313, 102.25) centre (-14.9313, 101.75) ccw
  line L247 (-14.4313, 101.75) -> (-14.4313, 88.75)
  arc A244 (-98.275, 31.1) -> (-97.775, 31.6) centre (-98.275, 31.6) ccw
  line L248 (-98.275, 31.1) -> (-111.275, 31.1)
  arc A245 (-111.775, 31.6) -> (-111.275, 31.1) centre (-111.275, 31.6) ccw
  line L249 (-111.775, 31.6) -> (-111.775, 44.6)
  arc A246 (-111.275, 45.1) -> (-111.775, 44.6) centre (-111.275, 44.6) ccw
  line L250 (-111.275, 45.1) -> (-98.275, 45.1)
  arc A247 (-97.775, 44.6) -> (-98.275, 45.1) centre (-98.275, 44.6) ccw
  line L251 (-97.775, 44.6) -> (-97.775, 31.6)
  arc A248 (-136.375, 31.1) -> (-135.875, 31.6) centre (-136.375, 31.6) ccw
  line L252 (-136.375, 31.1) -> (-149.375, 31.1)
  arc A249 (-149.875, 31.6) -> (-149.375, 31.1) centre (-149.375, 31.6) ccw
  line L253 (-149.875, 31.6) -> (-149.875, 44.6)
  arc A250 (-149.375, 45.1) -> (-149.875, 44.6) centre (-149.375, 44.6) ccw
  line L254 (-149.375, 45.1) -> (-136.375, 45.1)
  arc A251 (-135.875, 44.6) -> (-136.375, 45.1) centre (-136.375, 44.6) ccw
  line L255 (-135.875, 44.6) -> (-135.875, 31.6)
  arc A252 (-250.6752, 7.287) -> (-250.1752, 7.787) centre (-250.6752, 7.787) ccw
  line L256 (-250.6752, 7.287) -> (-263.6752, 7.287)
  arc A253 (-264.1753, 7.787) -> (-263.6752, 7.287) centre (-263.6752, 7.787) ccw
  line L257 (-264.1753, 7.787) -> (-264.1753, 20.787)
  arc A254 (-263.6752, 21.287) -> (-264.1753, 20.787) centre (-263.6752, 20.787) ccw
  line L258 (-263.6752, 21.287) -> (-250.6753, 21.287)
  arc A255 (-250.1753, 20.787) -> (-250.6753, 21.287) centre (-250.6753, 20.787) ccw
  line L259 (-250.1753, 20.787) -> (-250.1752, 7.787)
  arc A256 (-79.225, 7.287) -> (-78.725, 7.787) centre (-79.225, 7.787) ccw
  line L260 (-79.225, 7.287) -> (-92.225, 7.287)
  arc A257 (-92.725, 7.787) -> (-92.225, 7.287) centre (-92.225, 7.787) ccw
  line L261 (-92.725, 7.787) -> (-92.725, 20.787)
  arc A258 (-92.225, 21.287) -> (-92.725, 20.787) centre (-92.225, 20.787) ccw
  line L262 (-92.225, 21.287) -> (-79.225, 21.287)
  arc A259 (-78.725, 20.787) -> (-79.225, 21.287) centre (-79.225, 20.787) ccw
  line L263 (-78.725, 20.787) -> (-78.725, 7.787)
  arc A260 (-270.9156, 88.25) -> (-270.4156, 88.75) centre (-270.9156, 88.75) ccw
  line L264 (-270.9156, 88.25) -> (-283.9156, 88.25)
  arc A261 (-284.4156, 88.75) -> (-283.9156, 88.25) centre (-283.9156, 88.75) ccw
  line L265 (-284.4156, 88.75) -> (-284.4156, 101.75)
  arc A262 (-283.9156, 102.25) -> (-284.4156, 101.75) centre (-283.9156, 101.75) ccw
  line L266 (-283.9156, 102.25) -> (-270.9156, 102.25)
  arc A263 (-270.4156, 101.75) -> (-270.9156, 102.25) centre (-270.9156, 101.75) ccw
  line L267 (-270.4156, 101.75) -> (-270.4156, 88.75)
  arc A264 (-7.7875, 50.15) -> (-7.2875, 50.65) centre (-7.7875, 50.65) ccw
  line L268 (-7.7875, 50.15) -> (-20.7875, 50.15)
  arc A265 (-21.2875, 50.65) -> (-20.7875, 50.15) centre (-20.7875, 50.65) ccw
  line L269 (-21.2875, 50.65) -> (-21.2875, 63.65)
  arc A266 (-20.7875, 64.15) -> (-21.2875, 63.65) centre (-20.7875, 63.65) ccw
  line L270 (-20.7875, 64.15) -> (-7.7875, 64.15)
  arc A267 (-7.2875, 63.65) -> (-7.7875, 64.15) centre (-7.7875, 63.65) ccw
  line L271 (-7.2875, 63.65) -> (-7.2875, 50.65)
  arc A268 (-10.1687, 69.2) -> (-9.6687, 69.7) centre (-10.1687, 69.7) ccw
  line L272 (-10.1687, 69.2) -> (-23.1687, 69.2)
  arc A269 (-23.6687, 69.7) -> (-23.1687, 69.2) centre (-23.1688, 69.7) ccw
  line L273 (-23.6687, 69.7) -> (-23.6687, 82.7)
  arc A270 (-23.1687, 83.2) -> (-23.6687, 82.7) centre (-23.1688, 82.7) ccw
  line L274 (-23.1687, 83.2) -> (-10.1687, 83.2)
  arc A271 (-9.6687, 82.7) -> (-10.1687, 83.2) centre (-10.1688, 82.7) ccw
  line L275 (-9.6687, 82.7) -> (-9.6687, 69.7)
  arc A272 (-291.1562, 88.25) -> (-290.6563, 88.75) centre (-291.1563, 88.75) ccw
  line L276 (-291.1562, 88.25) -> (-304.1562, 88.25)
  arc A273 (-304.6562, 88.75) -> (-304.1563, 88.25) centre (-304.1563, 88.75) ccw
  line L277 (-304.6562, 88.75) -> (-304.6562, 101.75)
  arc A274 (-304.1562, 102.25) -> (-304.6562, 101.75) centre (-304.1563, 101.75) ccw
  line L278 (-304.1562, 102.25) -> (-291.1562, 102.25)
  arc A275 (-290.6562, 101.75) -> (-291.1562, 102.25) centre (-291.1562, 101.75) ccw
  line L279 (-290.6562, 101.75) -> (-290.6563, 88.75)
  arc A276 (-60.175, 31.1) -> (-59.675, 31.6) centre (-60.175, 31.6) ccw
  line L280 (-60.175, 31.1) -> (-73.175, 31.1)
  arc A277 (-73.675, 31.6) -> (-73.175, 31.1) centre (-73.175, 31.6) ccw
  line L281 (-73.675, 31.6) -> (-73.675, 44.6)
  arc A278 (-73.175, 45.1) -> (-73.675, 44.6) centre (-73.175, 44.6) ccw
  line L282 (-73.175, 45.1) -> (-60.175, 45.1)
  arc A279 (-59.675, 44.6) -> (-60.175, 45.1) centre (-60.175, 44.6) ccw
  line L283 (-59.675, 44.6) -> (-59.675, 31.6)
  arc A280 (-50.65, 50.15) -> (-50.15, 50.65) centre (-50.65, 50.65) ccw
  line L284 (-50.65, 50.15) -> (-63.65, 50.15)
  arc A281 (-64.15, 50.65) -> (-63.65, 50.15) centre (-63.65, 50.65) ccw
  line L285 (-64.15, 50.65) -> (-64.15, 63.65)
  arc A282 (-63.65, 64.15) -> (-64.15, 63.65) centre (-63.65, 63.65) ccw
  line L286 (-63.65, 64.15) -> (-50.65, 64.15)
  arc A283 (-50.15, 63.65) -> (-50.65, 64.15) centre (-50.65, 63.65) ccw
  line L287 (-50.15, 63.65) -> (-50.15, 50.65)
  arc A284 (-126.85, 50.15) -> (-126.35, 50.65) centre (-126.85, 50.65) ccw
  line L288 (-126.85, 50.15) -> (-139.85, 50.15)
  arc A285 (-140.35, 50.65) -> (-139.85, 50.15) centre (-139.85, 50.65) ccw
  line L289 (-140.35, 50.65) -> (-140.35, 63.65)
  arc A286 (-139.85, 64.15) -> (-140.35, 63.65) centre (-139.85, 63.65) ccw
  line L290 (-139.85, 64.15) -> (-126.85, 64.15)
  arc A287 (-126.35, 63.65) -> (-126.85, 64.15) centre (-126.85, 63.65) ccw
  line L291 (-126.35, 63.65) -> (-126.35, 50.65)
  arc A288 (-145.9001, 7.287) -> (-145.4001, 7.787) centre (-145.9001, 7.787) ccw
  line L292 (-145.9001, 7.287) -> (-158.9001, 7.287)
  arc A289 (-159.4001, 7.787) -> (-158.9001, 7.287) centre (-158.9001, 7.787) ccw
  line L293 (-159.4001, 7.787) -> (-159.4001, 20.787)
  arc A290 (-158.9001, 21.287) -> (-159.4001, 20.787) centre (-158.9001, 20.787) ccw
  line L294 (-158.9001, 21.287) -> (-145.9001, 21.287)
  arc A291 (-145.4001, 20.787) -> (-145.9001, 21.287) centre (-145.9001, 20.787) ccw
  line L295 (-145.4001, 20.787) -> (-145.4001, 7.787)
  arc A292 (-126.8501, 7.287) -> (-126.3501, 7.787) centre (-126.8501, 7.787) ccw
  line L296 (-126.8501, 7.287) -> (-139.8501, 7.287)
  arc A293 (-140.3501, 7.787) -> (-139.8501, 7.287) centre (-139.8501, 7.787) ccw
  line L297 (-140.3501, 7.787) -> (-140.3501, 20.787)
  arc A294 (-139.8501, 21.287) -> (-140.3501, 20.787) centre (-139.8501, 20.787) ccw
  line L298 (-139.8501, 21.287) -> (-126.8501, 21.287)
  arc A295 (-126.3501, 20.787) -> (-126.8501, 21.287) centre (-126.8501, 20.787) ccw
  line L299 (-126.3501, 20.787) -> (-126.3501, 7.787)
  arc A296 (-241.15, 50.15) -> (-240.65, 50.65) centre (-241.15, 50.65) ccw
  line L300 (-241.15, 50.15) -> (-254.15, 50.15)
  arc A297 (-254.65, 50.65) -> (-254.15, 50.15) centre (-254.15, 50.65) ccw
  line L301 (-254.65, 50.65) -> (-254.65, 63.65)
  arc A298 (-254.15, 64.15) -> (-254.65, 63.65) centre (-254.15, 63.65) ccw
  line L302 (-254.15, 64.15) -> (-241.15, 64.15)
  arc A299 (-240.65, 63.65) -> (-241.15, 64.15) centre (-241.15, 63.65) ccw